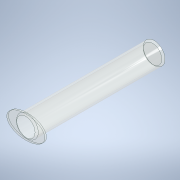
# Autodesk Inventor part: seringa outer
Saved by Autodesk Inventor 2021.2 (Build 252289000, 289)
## iProperties
Created: 2024-04-19
Part Number: seringa outer
Material: Glass
Document SubType Name: Modeling
Designer: cioba
Density: 2.18 g/cm^3
Appearance: Clear
Author: cioba
Autodesk Inventor part; units mm, degrees
ref_plane "YZ Plane" through (0, 0, 0) normal (1, 0, 0) x (0, 1, 0)
ref_plane "XZ Plane" through (0, 0, 0) normal (0, 1, 0) x (-1, 0, 0)
ref_plane "XY Plane" through (0, 0, 0) normal (0, 0, 1) x (1, 0, 0)
sketch "Sketch2" plane through (0, 0, 0) normal (0, 0, 1) x (1, 0, 0)
  circle A0 centre (-2.0274, 2.6474) radius 6.8
  ellipse E0 centre (-2.0274, 2.6474) end of major axis (-2.0274, -4.5526) minor radius 11.9605
  circle A1 centre (-2.0274, 2.6474) radius 5.8
  point P0 (0, 0)
  dimension "d25" = 1
  constraints: 2 centre point, 2 other
  measures "d25" radial gap between concentric circles of A0 A1
extrude "Extrusion5" add sketch "Sketch2" against normal blind 80.6 contours A0 | A1
extrude "Extrusion6" add sketch "Sketch2" against normal blind 1 contours E0
extrude "Extrusion7" cut sketch "Sketch2" against normal blind 79.6 contours A1
body "Solid3"
